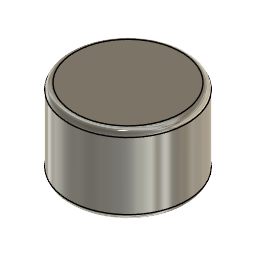
12_well_full_assembly (Autodesk Fusion 360 archive; units mm, degrees)
design "magnet"
Autodesk Fusion 360 part; units mm, degrees
sketch "Sketch1" plane through (0, 0, 0) normal (0, 0, 1) x (1, 0, 0)
  circle A0 centre (0, 0) radius 1.5
  dimension "d1" = 3
  constraint coincident A0.centre origin
  measures "d1" diameter of A0
extrude "Extrude1" add sketch "Sketch1" along normal blind 2
fillet "Fillet1" radius 0.15 2 edges at (-1.3985, -0.5424, 2) (-1.3985, -0.5424, 0)
